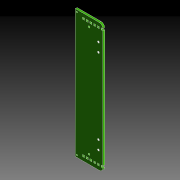
# Autodesk Inventor part: KB33-046-004-005 - Лицевая наклонная пластина
Saved by Autodesk Inventor 2020 (Build 240168000, 168)
## iProperties
Created: 2021-06-25
Part Number: KB33-046-004-005 - Лицевая наклонная пластина
Material: Типовые
Document SubType Name: Modeling
Designer: Петров Иван
Mass: 65.7241 g
Surface Area: 366.276 cm^2
Volume: 65.7241 cm^3
Density: 1 g/cm^3
Appearance: По умолчанию
Author: Петров Иван
Autodesk Inventor part; units mm, degrees
ref_plane "YZ Plane" through (0, 0, 0) normal (1, 0, 0) x (0, 1, 0)
ref_plane "XZ Plane" through (0, 0, 0) normal (0, 1, 0) x (-1, 0, 0)
ref_plane "XY Plane" through (0, 0, 0) normal (0, 0, 1) x (1, 0, 0)
sketch "Эскиз1" plane through (0, 0, 0) normal (0, 0, 1) x (1, 0, 0)
  circle A0 centre (3.6373, -247.3954) radius 1.5
  circle A1 centre (3.6373, 22.3954) radius 1.5 projected
  line L0 (0, 27) -> (60, 27)
  line L1 (60, 27) -> (60, -250.5454)
  line L2 (60, -250.5454) -> (0, -250.5454)
  line L3 (0, -250.5454) -> (0, 27)
  point P0 (0, 0)
  point P1 (0, -190.5454)
  dimension "d0" = 60
  dimension "d15" = 3.6373
  dimension "d16" = 3.15
  dimension "d17" = 277.5454
  constraints: 8 end point, 2 parallel, 1 centre point, 1 horizontal, 1 perpendicular, 2 other
  measures "d0" distance of L1.end L2.end
  measures "d15" distance from line of L3 A0.centre
  measures "d16" distance from line of L2 A0.centre
  measures "d17" distance of L0.end L1.end
extrude "Выдавливание1" add sketch "Эскиз1" along normal blind 4
thicken "Толщина1" operation add thickness 1.455 both sides no extend neighbours yes toward (0, -1, 0) faces at (20, -250.5454, 1.3333)
sketch "Эскиз2" plane through (0, 0, 4) normal (0, 0, 1) x (1, 0, 0)
  line L0 (60, 19) -> (56, 19)
  line L1 (56, 19) -> (56, 15)
  line L2 (56, 15) -> (60, 15)
  line L3 (60, 15) -> (60, 19)
  line L4 (60, -252.0004) -> (60, 27) projected
  line L5 (60, 27) -> (0, 27) projected
  point P0 (0, 0)
  dimension "d5" = 4
  dimension "d6" = 4
  dimension "d7" = 8
  constraints: 8 end point, 2 parallel, 1 horizontal, 1 perpendicular, 1 point on line
  measures "d5" distance of L2.end L1.end
  measures "d6" distance of L1.end L0.end
  measures "d7" distance between parallel lines of L5 L0
extrude "Выдавливание2" cut sketch "Эскиз2" against normal blind 10
pattern_linear "Прямоуг.массив1" count 6 spacing 8 along (-1, 0, 0) of "Выдавливание2"
ref_plane "РабПлоскость1" through (0, -112.5002, 4) normal (0, 1, 0) x (1, 0, 0)
mirror "Зеркальное отражение1" about plane through (0, -112.5002, 4) normal (0, 1, 0) of "Выдавливание2", "Прямоуг.массив1"
sketch "Эскиз3" plane through (0, 0, 4) normal (0, 0, 1) x (1, 0, 0)
  circle A0 centre (30, 7.5) radius 2
  circle A1 centre (30, -172.5) radius 2
  point P0 (0, 0)
  point P1 (0, 0)
  constraints: 2 centre point
extrude "Выдавливание3" cut sketch "Эскиз3" against normal blind 10 contours A0
mirror "Зеркальное отражение2" about plane through (0, -112.5002, 4) normal (0, 1, 0) of "Выдавливание3"
fillet "Сопряжение1" radius 8 2 edges at (60, 27, 2) (60, -252.0004, 2)
sketch "Эскиз4" plane through (0, 0, 0) normal (0, 0, -1) x (-1, 0, 0)
  circle A0 centre (-50.4709, -214.3241) radius 2 projected
  circle A1 centre (-50.4709, -194.8012) radius 2 projected
  circle A2 centre (-50.4709, -30.1988) radius 2 projected
  circle A3 centre (-50.4709, -10.6759) radius 2 projected
  point P0 (0, 0)
extrude "Выдавливание4" cut sketch "Эскиз4" against normal blind 10
